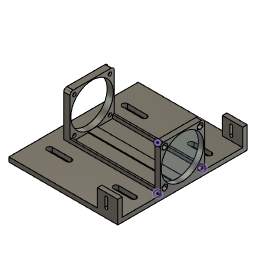
stepper caddy (Autodesk Fusion 360 design; units mm, degrees)
Autodesk Fusion 360 part; units mm, degrees
sketch "Sketch1" plane through (0, 0, 0) normal (0, 1, 0) x (1, 0, 0)
  line L0 (0, 0) -> (-120, 0)
  line L1 (-120, 0) -> (-120, -146)
  line L2 (-120, -146) -> (0, -146)
  line L3 (0, -146) -> (0, 0)
  dimension "d1" = 120
  dimension "d2" = 146
  constraint horizontal L0
  constraint vertical L1
  constraint horizontal L2
  constraint vertical L3
  constraint coincident L0.start L3.end
  measures "d1" distance of L0.start L0.end
  measures "d2" distance of L0.start L2.end
extrude "Extrude1" add sketch "Sketch1" along normal blind 5 makes body 1
sketch "Sketch2" plane through (0, 5, 0) normal (0, 1, 0) x (-1, 0, 0)
  line L0 (0, 146) -> (0, 0)
  line L1 (0, 0) -> (120, 0)
  line L2 (120, 0) -> (120, 146)
  line L3 (120, 146) -> (0, 146)
  line L4 (0, 0) -> (20, 0)
  line L5 (20, 0) -> (20, 5)
  line L6 (20, 5) -> (0, 5)
  line L7 (0, 5) -> (0, 0)
  dimension "d5" = 20
  dimension "d6" = 5
  constraint horizontal L4
  constraint vertical L5
  constraint horizontal L6
  constraint vertical L7
  constraint coincident L0.end L1.start
  measures "d5" distance of L0.end L4.end
  measures "d6" distance of L0.end L6.end
extrude "Extrude2" add sketch "Sketch2" along normal blind 20 contours L0 L1 L4 L5 L6 L7 bodies 1
sketch "Sketch3" plane through (0, 5, 0) normal (0, 1, 0) x (-1, 0, 0)
  line L0 (20, 5) -> (20, 0)
  line L1 (20, 0) -> (120, 0)
  line L2 (120, 0) -> (120, 146)
  line L3 (120, 146) -> (0, 146)
  line L4 (0, 146) -> (0, 5)
  line L5 (0, 5) -> (20, 5)
  line L6 (0, 146) -> (20, 146)
  line L7 (20, 146) -> (20, 141)
  line L8 (20, 141) -> (0, 141)
  line L9 (0, 141) -> (0, 146)
  dimension "d9" = 20
  dimension "d10" = 5
  constraint horizontal L6
  constraint vertical L7
  constraint horizontal L8
  constraint vertical L9
  constraint coincident L3.end L4.start
  measures "d9" distance of L3.end L6.end
  measures "d10" distance of L3.end L8.end
extrude "Extrude3" add sketch "Sketch3" along normal blind 20 contours L3 L4 L6 L7 L8 L9 bodies 1
sketch "Sketch4" plane through (0, 0, 146) normal (0, 0, 1) x (1, 0, 0)
  line L0 (-120, 0) -> (0, 0)
  line L1 (0, 0) -> (0, 25)
  line L2 (0, 25) -> (-20, 25)
  line L3 (-20, 25) -> (-20, 5)
  line L4 (-20, 5) -> (-120, 5)
  line L5 (-120, 5) -> (-120, 0)
  circle A0 centre (-10, 20) radius 1.55
  circle A1 centre (-10, 10) radius 1.55
  line L6 (-11.5495, 10.0376) -> (-11.55, 19.9999)
  line L7 (-8.4505, 10.0376) -> (-8.45, 19.9999)
  dimension "d13" = 3.1
  dimension "d14" = 3.1
  constraint coincident A1 L6.start
  constraint coincident A0 L6.end
  constraint tangent A0 L6
  constraint coincident A1 L7.start
  constraint coincident A0 L7.end
  constraint tangent A0 L7
  measures "d13" diameter of A0
  measures "d14" diameter of A1
extrude "Extrude4" cut sketch "Sketch4" against normal blind 300 contours A0 | A0 A1 L6 L7 | A1 bodies 1
sketch "Sketch5" plane through (0, 5, 0) normal (0, 1, 0) x (-1, 0, 0)
  line L0 (20, 146) -> (20, 141)
  line L1 (20, 141) -> (0, 141)
  line L2 (0, 141) -> (0, 5)
  line L3 (0, 5) -> (20, 5)
  line L4 (20, 5) -> (20, 0)
  line L5 (20, 0) -> (120, 0)
  line L6 (120, 0) -> (120, 146)
  line L7 (120, 146) -> (20, 146)
  line L8 (0, 5) -> (120, 5)
  line L9 (120, 5) -> (120, 20)
  line L10 (120, 20) -> (0, 20)
  line L11 (0, 20) -> (0, 5)
  line L12 (0, 20) -> (100, 20)
  line L13 (100, 20) -> (100, 48)
  line L14 (100, 48) -> (0, 48)
  line L15 (0, 48) -> (0, 20)
  line L16 (0, 48) -> (100, 48)
  line L17 (100, 48) -> (100, 98)
  line L18 (100, 98) -> (0, 98)
  line L19 (0, 98) -> (0, 48)
  line L20 (0, 98) -> (95, 98)
  line L21 (95, 126) -> (0, 126)
  line L22 (0, 126) -> (0, 98)
  circle A0 centre (10, 30) radius 3
  circle A1 centre (30, 30) radius 3
  line L23 (30, 33) -> (10, 33)
  line L24 (30, 27) -> (10, 27)
  line L25 (95, 126) -> (100, 126)
  line L26 (100, 126) -> (100, 70)
  line L27 (100, 70) -> (95, 70)
  circle A2 centre (95, 30) radius 3
  circle A3 centre (83, 30) radius 3
  line L28 (95, 27) -> (83, 27)
  line L29 (95, 33) -> (83, 33)
  circle A4 centre (10, 115) radius 3
  circle A5 centre (30, 115) radius 3
  line L30 (30, 112) -> (10, 112)
  line L31 (30, 118) -> (10, 118)
  circle A6 centre (95, 115) radius 3
  circle A7 centre (83, 115) radius 3
  line L32 (95, 112) -> (83, 112)
  line L33 (95, 118) -> (83, 118)
  circle A8 centre (105, 30) radius 3
  circle A9 centre (105, 115) radius 3
  line L34 (83, 118) -> (105, 118)
  line L35 (105, 112) -> (83, 112)
  line L36 (105, 27) -> (83, 27)
  line L37 (105, 33) -> (83, 33)
  dimension "d17" = 15
  dimension "d18" = 28
  dimension "d19" = 50
  dimension "d21" = 28
  constraint horizontal L8
  constraint vertical L9
  constraint horizontal L10
  constraint vertical L11
  constraint coincident L2.end L3.start
  constraint horizontal L12
  constraint vertical L13
  constraint horizontal L14
  constraint vertical L15
  constraint horizontal L16
  constraint vertical L17
  constraint horizontal L18
  constraint vertical L19
  constraint horizontal L20
  constraint horizontal L21
  constraint vertical L22
  constraint coincident A1 L23.start
  constraint coincident A0 L23.end
  constraint tangent A0 L23
  constraint horizontal L23
  constraint coincident A1 L24.start
  constraint coincident A0 L24.end
  constraint tangent A0 L24
  constraint parallel L23 L24
  constraint horizontal L25
  constraint vertical L26
  constraint horizontal L27
  constraint coincident L17 L26.end
  constraint coincident A2 L28.start
  constraint coincident A3 L28.end
  constraint tangent A3 L28
  constraint perpendicular L17 L28
  constraint coincident A2 L29.start
  constraint coincident A3 L29.end
  constraint tangent A3 L29
  constraint parallel L28 L29
  constraint coincident A5 L30.start
  constraint coincident A4 L30.end
  constraint tangent A4 L30
  constraint horizontal L30
  constraint coincident A5 L31.start
  constraint coincident A4 L31.end
  constraint tangent A4 L31
  constraint parallel L30 L31
  constraint coincident A6 L32.start
  constraint coincident A7 L32.end
  constraint tangent A7 L32
  constraint perpendicular L26 L32
  constraint coincident A6 L33.start
  constraint coincident A7 L33.end
  constraint tangent A7 L33
  constraint parallel L21 L33
  constraint coincident A9 L34.end
  constraint tangent A9 L34
  constraint perpendicular L26 L34
  constraint coincident A9 L35.start
  constraint coincident L32 L35.end
  constraint tangent A7 L35
  constraint coincident A8 L36.start
  constraint tangent A3 L36
  constraint coincident A8 L37.start
  constraint tangent A3 L37
  measures "d17" distance of L2.end L10.end
  measures "d18" distance of L10.end L14.end
  measures "d19" distance of L14.end L18.end
  measures "d21" distance of L18.end L21.end
extrude "Extrude5" cut sketch "Sketch5" against normal blind 40 contours L13 A2 L36 L37 | L13 A8 L36 L37 | A8 | A2 A3 L28 L29 L36 L37 | A2 | L26 A9 L34 L35 | L26 A6 L34 L35 | A3 | A6 | A6 A7 L32 L33 L34 L35 | A9 | A7 | A0 | A0 A1 L23 L24 | A1 | A4 | A4 A5 L30 L31 | A5 bodies 1
sketch "Sketch6" plane through (0, 5, 0) normal (0, 1, 0) x (-1, 0, 0)
  line L0 (83, 33) -> (105, 33)
  arc A0 (105, 27) -> (105, 33) centre (105, 30) ccw
  line L1 (105, 27) -> (83, 27)
  arc A1 (83, 33) -> (83, 27) centre (83, 30) ccw
  arc A2 (10, 33) -> (10, 27) centre (10, 30) ccw
  line L2 (10, 33) -> (30, 33)
  arc A3 (30, 27) -> (30, 33) centre (30, 30) ccw
  line L3 (30, 27) -> (10, 27)
  line L4 (105, 112) -> (83, 112)
  arc A4 (83, 118) -> (83, 112) centre (83, 115) ccw
  line L5 (83, 118) -> (105, 118)
  arc A5 (105, 112) -> (105, 118) centre (105, 115) ccw
  line L6 (10, 118) -> (30, 118)
  arc A6 (30, 112) -> (30, 118) centre (30, 115) ccw
  line L7 (30, 112) -> (10, 112)
  arc A7 (10, 118) -> (10, 112) centre (10, 115) ccw
  line L8 (20, 146) -> (20, 141)
  line L9 (20, 141) -> (0, 141)
  line L10 (0, 141) -> (0, 5)
  line L11 (0, 5) -> (20, 5)
  line L12 (20, 5) -> (20, 0)
  line L13 (20, 0) -> (120, 0)
  line L14 (120, 0) -> (120, 146)
  line L15 (120, 146) -> (20, 146)
  line L16 (0, 5) -> (15, 5)
  line L17 (15, 5) -> (15, 48)
  line L18 (15, 48) -> (0, 48)
  line L19 (0, 48) -> (0, 5)
  line L20 (0, 48) -> (3, 48)
  line L21 (3, 48) -> (3, 98)
  line L22 (3, 98) -> (0, 98)
  line L23 (0, 98) -> (0, 48)
  dimension "d24" = 43
  dimension "d25" = 3
  dimension "d26" = 50
  constraint horizontal L16
  constraint vertical L17
  constraint horizontal L18
  constraint vertical L19
  constraint coincident L10.end L11.start
  constraint horizontal L20
  constraint vertical L21
  constraint horizontal L22
  constraint vertical L23
  measures "d24" distance of L10.end L18.end
  measures "d25" distance of L18.end L20.end
  measures "d26" distance of L18.end L22.end
extrude "Extrude6" add sketch "Sketch6" along normal blind 50 contours L10 L18 L20 L21 L22 L23 bodies 1
sketch "Sketch7" plane through (0, 0, 0) normal (1, 0, 0) x (0, 0, -1)
  line L0 (-146, 0) -> (0, 0)
  line L1 (0, 0) -> (0, 25)
  line L2 (0, 25) -> (-5, 25)
  line L3 (-5, 25) -> (-5, 5)
  line L4 (-5, 5) -> (-48, 5)
  line L5 (-48, 5) -> (-48, 55)
  line L6 (-48, 55) -> (-98, 55)
  line L7 (-98, 55) -> (-98, 5)
  line L8 (-98, 5) -> (-141, 5)
  line L9 (-141, 5) -> (-141, 25)
  line L10 (-141, 25) -> (-146, 25)
  line L11 (-146, 25) -> (-146, 0)
  circle A0 centre (-73, 30.0634) radius 24.0001
sketch "Sketch8" plane through (0, 5, 0) normal (0, 1, 0) x (-1, 0, 0)
  line L0 (3, 48) -> (0, 48)
  line L1 (0, 48) -> (0, 5)
  line L2 (0, 5) -> (20, 5)
  line L3 (20, 5) -> (20, 0)
  line L4 (20, 0) -> (120, 0)
  line L5 (120, 0) -> (120, 146)
  line L6 (120, 146) -> (20, 146)
  line L7 (20, 146) -> (20, 141)
  line L8 (20, 141) -> (0, 141)
  line L9 (0, 141) -> (0, 98)
  line L10 (0, 98) -> (3, 98)
  line L11 (3, 98) -> (3, 48)
  line L12 (83, 33) -> (105, 33)
  arc A0 (105, 27) -> (105, 33) centre (105, 30) ccw
  line L13 (105, 27) -> (83, 27)
  arc A1 (83, 33) -> (83, 27) centre (83, 30) ccw
  arc A2 (10, 33) -> (10, 27) centre (10, 30) ccw
  line L14 (10, 33) -> (30, 33)
  arc A3 (30, 27) -> (30, 33) centre (30, 30) ccw
  line L15 (30, 27) -> (10, 27)
  line L16 (105, 112) -> (83, 112)
  arc A4 (83, 118) -> (83, 112) centre (83, 115) ccw
  line L17 (83, 118) -> (105, 118)
  arc A5 (105, 112) -> (105, 118) centre (105, 115) ccw
  line L18 (10, 118) -> (30, 118)
  arc A6 (30, 112) -> (30, 118) centre (30, 115) ccw
  line L19 (30, 112) -> (10, 112)
  arc A7 (10, 118) -> (10, 112) centre (10, 115) ccw
  line L20 (3, 98) -> (99, 98)
  line L21 (99, 98) -> (99, 48)
  line L22 (99, 48) -> (3, 48)
  line L23 (3, 48) -> (3, 98)
  line L24 (99, 98) -> (102, 98)
  line L25 (102, 98) -> (102, 48)
  line L26 (102, 48) -> (99, 48)
  line L27 (99, 48) -> (99, 98)
  dimension "d29" = 96
  dimension "d30" = 50
  dimension "d31" = 3
  dimension "d32" = 50
  constraint horizontal L20
  constraint vertical L21
  constraint horizontal L22
  constraint vertical L23
  constraint coincident L10.end L11.start
  constraint horizontal L24
  constraint vertical L25
  constraint horizontal L26
  constraint vertical L27
  measures "d29" distance of L10.end L20.end
  measures "d30" distance of L10.end L0.start
  measures "d31" distance of L20.end L24.end
  measures "d32" distance of L20.end L21.end
extrude "Extrude7" add sketch "Sketch8" along normal blind 50 contours L21 L24 L25 L26 L27 bodies 1
extrude "Extrude8" cut sketch "Sketch7" against normal blind 400 contours A0 bodies 1
sketch "Sketch9" plane through (0, 0, 0) normal (1, 0, 0) x (0, 0, -1)
  circle A0 centre (-73, 30.0634) radius 24.0001
  line L0 (-146, 0) -> (0, 0)
  line L1 (0, 0) -> (0, 25)
  line L2 (0, 25) -> (-5, 25)
  line L3 (-5, 25) -> (-5, 5)
  line L4 (-5, 5) -> (-48, 5)
  line L5 (-98, 5) -> (-141, 5)
  line L6 (-141, 5) -> (-141, 25)
  line L7 (-141, 25) -> (-146, 25)
  line L8 (-146, 25) -> (-146, 0)
sketch "Sketch10" plane through (0, 0, 0) normal (1, 0, 0) x (0, 0, -1)
  line L0 (-56, 48.2679) -> (-53, 46.5359)
  line L1 (-53, 46.5359) -> (-50, 48.2679)
  line L2 (-50, 48.2679) -> (-50, 51.7321)
  line L3 (-50, 51.7321) -> (-53, 53.4641)
  line L4 (-53, 53.4641) -> (-56, 51.7321)
  line L5 (-56, 51.7321) -> (-56, 48.2679)
  line L6 (-90, 51.7321) -> (-93, 53.4641)
  line L7 (-93, 53.4641) -> (-96, 51.7321)
  line L8 (-96, 51.7321) -> (-96, 48.2679)
  line L9 (-96, 48.2679) -> (-93, 46.5359)
  line L10 (-93, 46.5359) -> (-90, 48.2679)
  line L11 (-90, 48.2679) -> (-90, 51.7321)
  line L12 (-90, 11.7321) -> (-93, 13.4641)
  line L13 (-93, 13.4641) -> (-96, 11.7321)
  line L14 (-96, 11.7321) -> (-96, 8.2679)
  line L15 (-96, 8.2679) -> (-93, 6.5359)
  line L16 (-93, 6.5359) -> (-90, 8.2679)
  line L17 (-90, 8.2679) -> (-90, 11.7321)
  line L18 (-56, 8.2679) -> (-53, 6.5359)
  line L19 (-53, 6.5359) -> (-50, 8.2679)
  line L20 (-50, 8.2679) -> (-50, 11.7321)
  line L21 (-50, 11.7321) -> (-53, 13.4641)
  line L22 (-53, 13.4641) -> (-56, 11.7321)
  line L23 (-56, 11.7321) -> (-56, 8.2679)
  circle A0 centre (-53, 10) radius 2
  circle A1 centre (-93, 10) radius 2
  circle A2 centre (-93, 50) radius 2
  circle A3 centre (-53, 50) radius 2
  point P0 (-53, 50)
  point P1 (-93, 50)
  point P2 (-93, 10)
  point P3 (-53, 10)
  constraint coincident P3 A0.centre
  constraint coincident P2 A1.centre
  constraint coincident P1 A2.centre
  constraint coincident P0 A3.centre
extrude "Extrude9" cut sketch "Sketch10" against normal blind 900 contours A0 | A1 | A2 | A3 bodies 1
sketch "Sketch11" plane through (0, 0, 0) normal (1, 0, 0) x (0, 0, -1)
  line L0 (-90, 11.7321) -> (-93, 13.4641)
  line L1 (-93, 13.4641) -> (-96, 11.7321)
  line L2 (-96, 11.7321) -> (-96, 8.2679)
  line L3 (-96, 8.2679) -> (-93, 6.5359)
  line L4 (-93, 6.5359) -> (-90, 8.2679)
  line L5 (-90, 8.2679) -> (-90, 11.7321)
  circle A0 centre (-93, 10) radius 2
  line L6 (-56, 8.2679) -> (-53, 6.5359)
  line L7 (-53, 6.5359) -> (-50, 8.2679)
  line L8 (-50, 8.2679) -> (-50, 11.7321)
  line L9 (-50, 11.7321) -> (-53, 13.4641)
  line L10 (-53, 13.4641) -> (-56, 11.7321)
  line L11 (-56, 11.7321) -> (-56, 8.2679)
  circle A1 centre (-53, 10) radius 2
  line L12 (-56, 48.2679) -> (-53, 46.5359)
  line L13 (-53, 46.5359) -> (-50, 48.2679)
  line L14 (-50, 48.2679) -> (-50, 51.7321)
  line L15 (-50, 51.7321) -> (-53, 53.4641)
  line L16 (-53, 53.4641) -> (-56, 51.7321)
  line L17 (-56, 51.7321) -> (-56, 48.2679)
  circle A2 centre (-53, 50) radius 2
  line L18 (-90, 51.7321) -> (-93, 53.4641)
  line L19 (-93, 53.4641) -> (-96, 51.7321)
  line L20 (-96, 51.7321) -> (-96, 48.2679)
  line L21 (-96, 48.2679) -> (-93, 46.5359)
  line L22 (-93, 46.5359) -> (-90, 48.2679)
  line L23 (-90, 48.2679) -> (-90, 51.7321)
  circle A3 centre (-93, 50) radius 2
  point P0 (-93, 10)
  point P1 (-53, 10)
  point P2 (-53, 50)
  point P3 (-93, 50)
  constraint coincident P0 A0.centre
  constraint coincident P1 A1.centre
  constraint coincident P2 A2.centre
  constraint coincident P3 A3.centre
extrude "Extrude10" cut sketch "Sketch11" against normal blind 1 bodies 1
sketch "Sketch12" plane through (-102, 0, 0) normal (-1, 0, 0) x (0, 0, 1)
  circle A0 centre (53, 50) radius 2
  circle A1 centre (53, 10) radius 2
  circle A2 centre (93, 50) radius 2
  circle A3 centre (93, 10) radius 2
  circle A4 centre (73, 30.0634) radius 24.0001
  line L0 (48, 5) -> (98, 5)
  line L1 (98, 5) -> (98, 55)
  line L2 (98, 55) -> (48, 55)
  line L3 (48, 55) -> (48, 5)
  line L4 (56, 51.7321) -> (53, 53.4641)
  line L5 (53, 53.4641) -> (50, 51.7321)
  line L6 (50, 51.7321) -> (50, 48.2679)
  line L7 (50, 48.2679) -> (53, 46.5359)
  line L8 (53, 46.5359) -> (56, 48.2679)
  line L9 (56, 48.2679) -> (56, 51.7321)
  line L10 (96, 51.7321) -> (93, 53.4641)
  line L11 (93, 53.4641) -> (90, 51.7321)
  line L12 (90, 51.7321) -> (90, 48.2679)
  line L13 (90, 48.2679) -> (93, 46.5359)
  line L14 (93, 46.5359) -> (96, 48.2679)
  line L15 (96, 48.2679) -> (96, 51.7321)
  line L16 (90, 8.2679) -> (93, 6.5359)
  line L17 (93, 6.5359) -> (96, 8.2679)
  line L18 (96, 8.2679) -> (96, 11.7321)
  line L19 (96, 11.7321) -> (93, 13.4641)
  line L20 (93, 13.4641) -> (90, 11.7321)
  line L21 (90, 11.7321) -> (90, 8.2679)
  line L22 (56, 11.7321) -> (53, 13.4641)
  line L23 (53, 13.4641) -> (50, 11.7321)
  line L24 (50, 11.7321) -> (50, 8.2679)
  line L25 (50, 8.2679) -> (53, 6.5359)
  line L26 (53, 6.5359) -> (56, 8.2679)
  line L27 (56, 8.2679) -> (56, 11.7321)
  point P0 (53, 50)
  point P1 (93, 50)
  point P2 (93, 10)
  point P3 (53, 10)
  constraint coincident P0 A0.centre
  constraint coincident P1 A2.centre
  constraint coincident P2 A3.centre
  constraint coincident P3 A1.centre
extrude "Extrude11" cut sketch "Sketch12" against normal blind 1 contours L4 L5 L6 L7 L8 L9 | L10 L11 L12 L13 L14 L15 | L16 L17 L18 L19 L20 L21 | L22 L23 L24 L25 L26 L27 bodies 1
copy_body "Body->Comp1" bodies 1 removing the originals makes body 2 in component "Component"
sketch "Sketch13" plane through (0, 0, 0) normal (0, 1, 0) x (1, 0, 0)
extrude "Extrude1'" add 1 faces at (-102, 44.1092, 94.4844) along direction (-1, 0, 0) blind 4 on bodies 2 bodies 2 in component "Component"
sketch "Sketch14" plane through (0, 0, 0) normal (1, 0, 0) x (0, 0, -1)
  point P0 (-98, 5)
  point P1 (-48, 5)
  point P2 (-98, 55)
extrude "Extrude2'" add 1 faces at (0, 1.6667, 81.3333) along direction (1, 0, 0) blind 3 on bodies 2 bodies 2 in component "Component"
sketch "Sketch15" plane through (-99, 0, 0) normal (1, 0, 0) x (0, 0, -1)
  circle A0 centre (-53, 50) radius 2
  circle A1 centre (-53, 10) radius 2
  circle A2 centre (-93, 50) radius 2
  circle A3 centre (-93, 10) radius 2
  circle A4 centre (-73, 30.0634) radius 24.0001
  line L0 (-98, 5) -> (-48, 5)
  line L1 (-48, 5) -> (-48, 55)
  line L2 (-48, 55) -> (-98, 55)
  line L3 (-98, 55) -> (-98, 5)
  line L4 (-98, 5) -> (-96, 5)
  line L5 (-96, 5) -> (-96, 9)
  line L6 (-96, 9) -> (-98, 9)
  line L7 (-98, 9) -> (-98, 5)
  constraint horizontal L4
  constraint vertical L5
  constraint horizontal L6
  constraint vertical L7
  constraint coincident L0.start L3.end
extrude "Extrude3'" add sketch "Sketch15" along normal blind 96 contours L0 L3 L4 L5 L6 L7 bodies 2 in component "Component"
sketch "Sketch16" plane through (-3, 0, 0) normal (-1, 0, 0) x (0, 0, 1)
  line L0 (96, 9) -> (98, 9)
  line L1 (98, 9) -> (98, 55)
  line L2 (98, 55) -> (48, 55)
  line L3 (48, 55) -> (48, 5)
  line L4 (48, 5) -> (96, 5)
  line L5 (96, 5) -> (96, 9)
  circle A0 centre (53, 50) radius 2
  circle A1 centre (53, 10) radius 2
  circle A2 centre (93, 50) radius 2
  circle A3 centre (93, 10) radius 2
  circle A4 centre (73, 30.0634) radius 24.0001
  line L6 (48, 5) -> (50, 5)
  line L7 (50, 5) -> (50, 9)
  line L8 (50, 9) -> (48, 9)
  line L9 (48, 9) -> (48, 5)
  constraint horizontal L6
  constraint vertical L7
  constraint horizontal L8
  constraint vertical L9
  constraint coincident L3.end L4.start
extrude "Extrude4'" add sketch "Sketch16" along normal blind 96 contours L3 L4 L6 L7 L8 L9 bodies 2 in component "Component"
sketch "Sketch17" plane through (-3, 0, 0) normal (-1, 0, 0) x (0, 0, 1)
  line L0 (50, 9) -> (50, 5)
  line L1 (50, 5) -> (96, 5)
  line L2 (96, 5) -> (96, 9)
  line L3 (96, 9) -> (98, 9)
  line L4 (98, 9) -> (98, 55)
  line L5 (98, 55) -> (48, 55)
  line L6 (48, 55) -> (48, 9)
  line L7 (48, 9) -> (50, 9)
  circle A0 centre (53, 50) radius 2
  circle A1 centre (53, 10) radius 2
  circle A2 centre (93, 50) radius 2
  circle A3 centre (93, 10) radius 2
  circle A4 centre (73, 30.0634) radius 24.0001
  line L8 (77.5404, 5) -> (67.5, 5)
  line L9 (67.5, 5) -> (67.5, 6)
  line L10 (67.5, 6) -> (77.5404, 6)
  line L11 (77.5404, 6) -> (77.5404, 5)
  constraint horizontal L8
  constraint vertical L9
  constraint horizontal L10
  constraint vertical L11
  constraint coincident L1 L8.start
extrude "Extrude5'" add sketch "Sketch17" along normal blind 96 contours L1 L8 L9 L10 L11 bodies 2 in component "Component"
fillet "Fillet1" radius 3.5 1 edges at (0, 55, 48) on bodies 2 in component "Component"
fillet "Fillet2" radius 3.5 1 edges at (0, 55, 98) on bodies 2 in component "Component"
fillet "Fillet3" radius 3.5 1 edges at (-102.5, 55, 98) on bodies 2 in component "Component"
fillet "Fillet4" radius 3.5 1 edges at (-102.5, 55, 48) on bodies 2 in component "Component"
fillet "Fillet5" radius 1 1 edges at (-120, 0, 73) on bodies 2 in component "Component"
component "Component" placed x (1, 0, 0) y (0, 1, 0) z (0, 0, 1) at (0, 0, 0)
